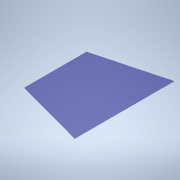
# Autodesk Inventor part: Measuringrange_OXS200_11728845
Saved by Autodesk Inventor 2021 (Build 250183000, 183)
## iProperties
Created: 2025-06-20
Part Number: Measuringrange_OXS200_11728845
Material: Generic
Catalog Web Link: www.cadenas.de
Description: ox_emerging_beam-emerging beam
Vendor: BAUMER
Document SubType Name: Modeling
Designer: psAdmin
Manufacturer: BAUMER
Mass: 13.6398 g
Surface Area: 239.214 cm^2
Volume: 13.6398 cm^3
Density: 1 g/cm^3
Appearance: PSOLRGB-0-0-255
Category: PARTsolutions
Company: BAUMER
Title: Measuringrange_OXS200_11728845
Author: Cadenas PARTsolutions
Comments: emerging beam
PSOL_IDENT_0: {$CADENAS_DATA/23d-libs/baumer/products/smartvisionsensors/smartprofilesensors/oxmp/oxmp_emerging_be
PSOL_IDENT_1: am.prj},211 {VTYP=3D},{NB=Measuringrange_OXS200_11728845},{LINA=Measuringrange_OXS200_11728845},{NN=
PSOL_IDENT_2: ox_emerging_beam},{DATE=12.06.2025 11:27:17},{GEOMDATE=06.05.2025 06:43:21},{VERSION=},{LINEID=350},
PSOL_IDENT_3: {WBVAR=},{WBNUMERIC=}  {NB=Measuringrange_OXS200_11728845},{LINA=Measuringrange_OXS200_11728845},{KT=
PSOL_IDENT_4: DUMMY},{TYPE=Measuring mode (E): Edge, Width/Gap, Intensity Edge, Segment Selector, Caliper X/Z/Dist
PSOL_IDENT_5: ance},{LWL=Red (660 nm)},{MR=100},{TC=OXS200-R10A.E02},{TCX=OXS200},{AN=11728845},{WS=icon_website.p
PSOL_IDENT_6: ng},{EP=eplan_data_standard.png},{MH=Aluminium},{MO=Glass},{WT=270},{PC=IP 65},{LC=2},{ET=18 … 30 VD
PSOL_IDENT_7: C},{AOS=4-20mA, 2-10mA, 0-10V, 0-5V},{SO=2 x Outputs (Push-Pull)},{CONS=typ. 2.4W (100 mA max at 24
PSOL_IDENT_8: V) | IEEE 802.3af Power over Ethernet (PoE)},{OT=0 ... + 45 °C},{ALI=< 25 kLux},{CS=CE, UL, PROFINET
PSOL_IDENT_9: , ETHERNET/IP},{EC=t.b.d.},{CTN=t.b.d.},{COO=t.b.d.},{TYPEX=1},{LWLX=1},{B0=7.800},{H0=3.000},{SDC=1
PSOL_IDENT_10: 50.000},{B1=75.000},{H1=0.650},{B2=144.400},{H2=0.750},{EH=8.500},{RH=37.300},{RW=12.000},{HX=0.400}
PSOL_IDENT_11: ,{L2=250.000}
NB: Measuringrange_OXS200_11728845
NN: ox_emerging_beam
NT: emerging beam
NBSYN: Measuringrange_$TCX._$AN.
LINA: Measuringrange_OXS200_11728845
CATALOG: Baumer Group
TYPE: Measuring mode (E): Edge, Width/Gap, Intensity Edge, Segment Selector, Caliper X/Z/Distance
LWL: Red (660 nm)
MR: 100
TC: OXS200-R10A.E02
TCX: OXS200
AN: 11728845
WS: icon_website.png
EP: eplan_data_standard.png
MH: Aluminium
MO: Glass
WT: 270
PC: IP 65
LC: 2
ET: 18 … 30 VDC
AOS: 4-20mA, 2-10mA, 0-10V, 0-5V
SO: 2 x Outputs (Push-Pull)
CONS: typ. 2.4W (100 mA max at 24 V) | IEEE 802.3af Power over Ethernet (PoE)
OT: 0 ... + 45 °C
ALI: < 25 kLux
CS: CE, UL, PROFINET, ETHERNET/IP
EC: t.b.d.
CTN: t.b.d.
COO: t.b.d.
HX: 0.4
L2: 250
SUPPLIER: BAUMER
ARTICLENO: Measuringrange_OXS200_11728845
BOMINFO: Measuringrange_OXS200_11728845
CREATOR: CADENAS GmbH
Autodesk Inventor part; units mm, degrees
sketch "Sketch_2" plane through (0, 0, 0) normal (1, 0, 0) x (0, 1, 0)
  line L0 (-1.5, 3.9) -> (-1.5, -3.9)
  line L1 (-1.5, -3.9) -> (1.5, -3.9)
  line L2 (1.5, -3.9) -> (1.5, 3.9)
  line L3 (1.5, 3.9) -> (-1.5, 3.9)
  constraints: 8 end point
sketch "Sketch_3" plane through (250, 0, 0) normal (1, 0, 0) x (0, 0, -1)
  line L0 (-72.2, -0.375) -> (72.2, -0.375)
  line L1 (72.2, -0.375) -> (72.2, 0.375)
  line L2 (72.2, 0.375) -> (-72.2, 0.375)
  line L3 (-72.2, 0.375) -> (-72.2, -0.375)
  constraints: 8 end point
loft "Loft1" add profiles "Sketch_2", "Sketch_3"
sketch "Sketch_4" plane through (0, 0, 0) normal (0, 0, 1) x (1, 0, 0)
  line L0 (0, 7.8) -> (0, -7.8)
  line L1 (0, -7.8) -> (150, -7.8)
  line L2 (150, -7.8) -> (150, 7.8)
  line L3 (150, 7.8) -> (0, 7.8)
  constraints: 8 end point
extrude "Extrusion1" cut sketch "Sketch_4" along normal mid plane 288.8
ref_plane "CP1_XY" through (0, 0, 0) normal (0, 0, 1) x (1, 0, 0)
ref_plane "CP1_YZ" through (0, 0, 0) normal (1, 0, 0) x (0, 1, 0)
ref_plane "CP1_ZX" through (0, 0, 0) normal (0, 1, 0) x (0, 0, 1)
body "Solid1"
